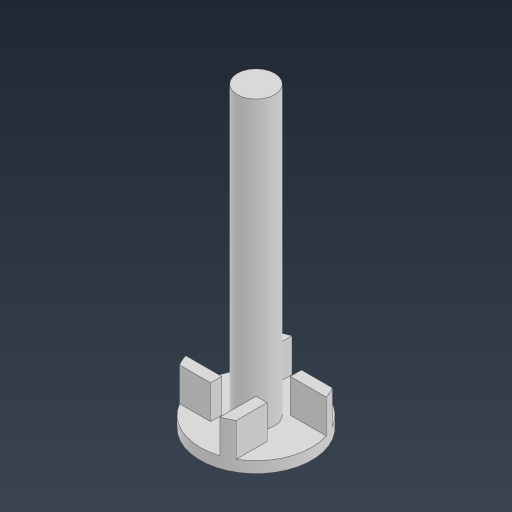
# Autodesk Inventor part: claw_nut
Saved by Autodesk Inventor 2023 (Build 270158000, 158)
## iProperties
Created: 2026-01-23
Part Number: claw_nut
Material: Generic
Document SubType Name: Modeling
Designer: szymo
Density: 1 g/cm^3
Appearance: Default
Author: szymo
Autodesk Inventor part; units mm, degrees
ref_plane "YZ Plane" through (0, 0, 0) normal (1, 0, 0) x (0, 1, 0)
ref_plane "XZ Plane" through (0, 0, 0) normal (0, 1, 0) x (-1, 0, 0)
ref_plane "XY Plane" through (0, 0, 0) normal (0, 0, 1) x (1, 0, 0)
sketch "Sketch1" plane through (0, 0, 0) normal (0, 1, 0) x (-1, 0, 0)
  circle A0 centre (0, 0) radius 7.5
  circle A1 centre (0, 0) radius 2.5
  dimension "d0" = 15
  dimension "d1" = 5
  constraints: 2 centre point, 2 coincident
  measures "d0" diameter of A0
  measures "d1" diameter of A1
extrude "Extrusion1" add sketch "Sketch1" along normal blind 1.5 contours A0 | A1
sketch "Sketch2" plane through (0, 1.5, 0) normal (0, 1, 0) x (1, 0, 0)
  circle A0 centre (0, 0) radius 2.5
  circle A1 centre (0, 0) radius 7.5 projected
  line L0 (-0.9798, 2.3) -> (-7.1386, 2.3)
  circle A2 centre (0, 0) radius 7.5 projected
  line L1 (-2.3, 0.9798) -> (-2.3, 7.1386)
  line L2 (-2.3, 7.1386) -> (-7.1386, 2.3)
  line L3 (-3.8, 2.3) -> (-3.8, 6.4661)
  line L4 (-2.3, -0.9798) -> (-2.3, -7.1386)
  line L5 (-0.9798, -2.3) -> (-7.1386, -2.3)
  line L6 (-2.3, -3.8) -> (-6.4661, -3.8)
  line L7 (-7.1386, -2.3) -> (-2.3, -7.1386)
  line L8 (0.9798, -2.3) -> (7.1386, -2.3)
  line L9 (2.3, -0.9798) -> (2.3, -7.1386)
  line L10 (3.8, -2.3) -> (3.8, -6.4661)
  line L11 (2.3, -7.1386) -> (7.1386, -2.3)
  line L12 (2.3, 0.9798) -> (2.3, 7.1386)
  line L13 (0.9798, 2.3) -> (7.1386, 2.3)
  line L14 (2.3, 3.8) -> (6.4661, 3.8)
  line L15 (7.1386, 2.3) -> (2.3, 7.1386)
  point P0 (2.3, -2.3)
  point P1 (2.3, -7.1386)
  point P2 (2.3, 2.3)
  point P3 (-2.3, 2.3)
  point P4 (-2.3, -2.3)
  dimension "d4" = 5
  dimension "d5" = 2.3
  dimension "d6" = 2.3
  dimension "d7" = 6.8429
  dimension "d8" = 1.5
  dimension "d11" = 360
  constraints: 32 end point, 5 point on circle, 4 point on line, 2 vertical, 1 centre point, 1 coincident, 1 horizontal, 41 other
  measures "d4" diameter of A0
  measures "d5" distance from line of L1 point (0, 0)
  measures "d6" distance from line of point (0, 0) L0
  measures "d7" distance of L1.end L0.end
  measures "d8" distance between parallel lines of L3 L1
extrude "Extrusion2" add sketch "Sketch2" along normal blind 4.5 contours L12 L14 L15 L13 | L8 L10 L11 L9 | L15 L14 A1 | L11 L10 A1 | L0 L3 L2 L1 | L4 L6 L7 L5 | L2 L3 A1 | L7 L6 A1 picked at (6.5762, 2.972) picked at (2.972, -6.5762) picked at (-2.972, 6.5762) picked at (-6.5762, -2.972)
sketch "Sketch3" plane through (0, 1.5, 0) normal (0, 1, 0) x (1, 0, 0)
  circle A0 centre (0, 0) radius 2.5
  dimension "d15" = 5
  constraints: 1 centre point, 1 coincident
  measures "d15" diameter of A0
extrude "Extrusion3" add sketch "Sketch3" along normal blind 38.5
sketch "Sketch4" plane through (0, 0, 0) normal (0, -1, 0) x (1, 0, 0)
  point P0 (0, 0)
  point P1 (0, 0)
  constraints: 1 coincident
hole "Hole1" [suppressed]
fillet "Fillet1" [suppressed]
equation "\"d6\" = d5"
body "Solid1"
